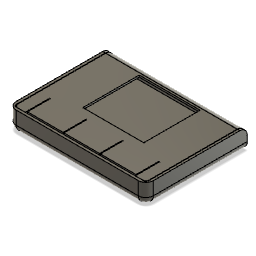
ProM Display Halter v12 (Autodesk Fusion 360 design; units mm, degrees)
Autodesk Fusion 360 part; units mm, degrees
note: some values were not read from the file. Set by a fixed rule: which sketch regions a step uses.
sketch "Skizze1" plane through (0, 0, 0) normal (0, 1, 0) x (1, 0, 0)
  line L0 (0, 0) -> (68, 0)
  line L1 (68, 0) -> (68, -48)
  line L2 (68, -48) -> (0, -48)
  line L3 (0, -48) -> (0, 0)
  line L4 (0, -48) -> (3.3, -48)
  line L5 (3.3, -48) -> (3.3, -33)
  line L6 (3.3, -33) -> (3.3, -20)
  circle A0 centre (3.3, -20) radius 2.5
  circle A1 centre (3.3, -33) radius 2.5
  line L7 (68, -48) -> (64.7, -48)
  line L8 (64.7, -48) -> (64.7, -33)
  line L9 (64.7, -33) -> (64.7, -20)
  circle A2 centre (64.7, -20) radius 2.5
  circle A3 centre (64.7, -33) radius 2.5
  dimension "d1" = 68
  dimension "d2" = 48
  dimension "d11" = 3.3
  dimension "d12" = 15
  dimension "d13" = 13
  dimension "d14" = 5
  dimension "d15" = 5
  dimension "d16" = 3.3
  dimension "d17" = 15
  dimension "d18" = 13
  dimension "d19" = 5
  dimension "d20" = 5
  constraint horizontal L0
  constraint vertical L1
  constraint horizontal L2
  constraint vertical L3
  constraint coincident L0.start L3.end
  constraint perpendicular L3 L4
  constraint perpendicular L4 L5
  constraint parallel L5 L6
  constraint coincident L6.end A0.centre
  constraint coincident L5.end L6.start
  constraint perpendicular L1 L7
  constraint vertical L8
  constraint perpendicular L2 L9
  constraint coincident L9.end A2.centre
  constraint coincident L8.end L9.start
  measures "d1" distance of L0.start L0.end
  measures "d2" distance of L0.start L2.end
  measures "d11" distance of L2.end L4.end
  measures "d12" distance of L4.end L5.end
  measures "d13" distance of L5.end L6.end
  measures "d14" diameter of A0
  measures "d15" diameter of A1
  measures "d16" distance of L1.end L7.end
  measures "d17" distance of L7.end L8.end
  measures "d18" distance of L8.end L9.end
  measures "d19" diameter of A2
  measures "d20" diameter of A3
extrude "Extrusion1" add sketch "Skizze1" along normal blind 1.2 makes body 1
move_body "Verschieben1" bodies 1 to x (1, 0, 0) y (0, 1, 0) z (0, 0, 1) at (0, 10, 0)
sketch "Skizze2" plane through (0, 0, 0) normal (0, 1, 0) x (1, 0, 0)
  line L0 (0, 0) -> (73, 0)
  line L1 (73, 0) -> (73, -54)
  line L2 (73, -54) -> (0, -54)
  line L3 (0, -54) -> (0, 0)
  dimension "d21" = 73
  dimension "d22" = 54
  constraint horizontal L0
  constraint vertical L1
  constraint horizontal L2
  constraint vertical L3
  constraint coincident L0.start L3.end
  measures "d21" distance of L0.start L0.end
  measures "d22" distance of L0.start L2.end
sketch "Skizze4" plane through (0, 0, 0) normal (0, 1, 0) x (1, 0, 0)
  line L0 (0, 0) -> (73, 0)
  line L1 (73, 0) -> (73, -54)
  line L2 (73, -54) -> (0, -54)
  line L3 (0, -54) -> (0, 0)
  line L4 (71.6, -1.4) -> (71.6, -52.6)
  line L5 (71.6, -52.6) -> (1.4, -52.6)
  line L6 (1.4, -52.6) -> (1.4, -1.4)
  line L7 (71, -2) -> (71, -52)
  line L8 (71, -52) -> (2, -52)
  line L9 (2, -52) -> (2, -2)
  line L10 (2, -2) -> (71, -2)
  line L11 (1.4, -1.4) -> (1.4, 0)
  line L12 (2, -2) -> (1.4, -2)
  line L13 (71.6, -1.4) -> (71.6, 0)
  line L14 (71, -2) -> (71.6, -2)
  line L15 (73, -24.3) -> (54, -24.3)
  line L16 (54, -24.3) -> (56.9, -24.3)
  circle A0 centre (56.9, -24.3) radius 2.9
  line L17 (56.9, -24.3) -> (56.9, 0)
  line L18 (56.9, -24.3) -> (73, -24.3)
  circle A1 centre (16.1, -24.3) radius 2.9
  line L19 (16.1, -24.3) -> (0, -24.3)
  line L20 (16.1, -24.3) -> (16.1, 0)
  line L21 (16.1, -24.3) -> (16.1, -40.5)
  circle A2 centre (16.1, -40.5) radius 2.9
  line L22 (56.9, -24.3) -> (56.9, -40.5)
  circle A3 centre (56.9, -40.5) radius 2.9
  line L23 (73, -23.8) -> (67.8, -23.8)
  line L24 (67.8, -23.8) -> (67.8, 0)
  circle A4 centre (67.8, -23.8) radius 2.5
  line L25 (67.8, -23.8) -> (67.8, -35.8)
  circle A5 centre (67.8, -35.8) radius 2.5
  line L26 (0, -23.8) -> (5.2, -23.8)
  line L27 (5.2, -23.8) -> (5.2, 0)
  circle A6 centre (5.2, -23.8) radius 2.5
  line L28 (5.2, -23.8) -> (5.2, -35.8)
  circle A7 centre (5.2, -35.8) radius 2.5
  circle A8 centre (5.2, -35.8) radius 1.4
  circle A9 centre (5.2, -23.8) radius 1.4
  circle A10 centre (67.8, -35.8) radius 1.4
  circle A11 centre (67.8, -23.8) radius 1.4
  circle A12 centre (56.9, -40.5) radius 1.1
  circle A13 centre (56.9, -24.3) radius 1.1
  circle A14 centre (16.1, -24.3) radius 1.1
  circle A15 centre (16.1, -40.5) radius 1.1
  dimension "d28" = 73
  dimension "d29" = 54
  dimension "d31" = 2
  dimension "d47" = 5.8
  dimension "d48" = 24.3
  dimension "d49" = 16.1
  dimension "d50" = 5.8
  dimension "d51" = 24.3
  dimension "d52" = 16.1
  dimension "d53" = 16.2
  dimension "d54" = 5.8
  dimension "d55" = 16.2
  dimension "d56" = 5.8
  dimension "d57" = 5.2
  dimension "d58" = 23.8
  dimension "d59" = 5
  dimension "d60" = 12
  dimension "d61" = 5
  dimension "d62" = 5.2
  dimension "d63" = 23.8
  dimension "d64" = 5
  dimension "d65" = 12
  dimension "d66" = 5
  dimension "d69" = 2.8
  dimension "d70" = 2.8
  dimension "d71" = 2.8
  dimension "d72" = 2.8
  dimension "d73" = 2.2
  dimension "d74" = 2.2
  dimension "d75" = 2.2
  dimension "d76" = 2.2
  constraint horizontal L0
  constraint vertical L1
  constraint horizontal L2
  constraint vertical L3
  constraint coincident L0.start L3.end
  constraint coincident L0 L11.end
  constraint perpendicular L0 L11
  constraint coincident L6 L12.end
  constraint perpendicular L6 L12
  constraint coincident L0 L13.end
  constraint perpendicular L0 L13
  constraint coincident L4 L14.end
  constraint perpendicular L4 L14
  constraint parallel L1 L4
  constraint parallel L2 L5
  constraint parallel L3 L6
  constraint coincident L1 L15.start
  constraint perpendicular L1 L15
  constraint parallel L15 L16
  constraint coincident L16.end A0.centre
  constraint coincident L0 L17.end
  constraint perpendicular L0 L17
  constraint coincident A1.centre L19.start
  constraint coincident L3 L19.end
  constraint perpendicular L3 L19
  constraint coincident L0 L20.end
  constraint perpendicular L0 L20
  constraint perpendicular L19 L21
  constraint coincident L21.end A2.centre
  constraint vertical L22
  constraint coincident L22.end A3.centre
  constraint coincident L1 L23.start
  constraint perpendicular L4 L23
  constraint coincident L0 L24.end
  constraint perpendicular L0 L24
  constraint coincident L23.end L24.start
  constraint perpendicular L18 L25
  constraint coincident L25.end A5.centre
  constraint coincident L3 L26.start
  constraint perpendicular L6 L26
  constraint coincident L0 L27.end
  constraint perpendicular L0 L27
  constraint coincident L26.end L27.start
  constraint perpendicular L26 L28
  constraint coincident L28.end A7.centre
  constraint concentric A7 A8
  constraint concentric A6 A9
  constraint concentric A5 A10
  constraint concentric A4 A11
  constraint concentric A3 A12
  constraint concentric A0 A13
  constraint concentric A1 A14
  constraint concentric A2 A15
  measures "d28" distance of L0.start L0.end
  measures "d29" distance of L0.start L2.end
  measures "d47" diameter of A0
  measures "d48" distance of L16.end L17.end
  measures "d49" distance of L15.start L16.end
  measures "d50" diameter of A1
  measures "d51" distance of A1.centre L20.end
  measures "d52" distance of A1.centre L19.end
  measures "d53" distance of A1.centre L21.end
  measures "d54" diameter of A2
  measures "d55" distance of L16.end L22.end
  measures "d56" diameter of A3
  measures "d57" distance of L23.start L23.end
  measures "d58" distance of L23.end L24.end
  measures "d59" diameter of A4
  measures "d60" distance of L23.end L25.end
  measures "d61" diameter of A5
  measures "d62" distance of L26.start L26.end
  measures "d63" distance of L26.end L27.end
  measures "d64" diameter of A6
  measures "d65" distance of L26.end L28.end
  measures "d66" diameter of A7
  measures "d69" diameter of A8
  measures "d70" diameter of A9
  measures "d71" diameter of A10
  measures "d72" diameter of A11
  measures "d73" diameter of A12
  measures "d74" diameter of A13
  measures "d75" diameter of A14
  measures "d76" diameter of A15
extrude "Extrusion7" add sketch "Skizze4" along normal blind 5 separate body contours L19 L27 A6 A9 | L26 L27 A6 A9 | L19 L26 A6 A9 | A1 L19 L20 A14 | A1 L20 L21 A14 | L19 A6 L28 A9 | L15 L16 A0 L17 A13 | L15 A0 L17 L18 A13 | A1 L19 L21 A14 | L19 A6 L28 A9 | L23 L24 A4 A11 | L15 L18 L24 A4 A11 | L15 A0 L18 L22 A13 | L15 L16 A0 L22 A13 | L15 L18 L23 A4 A11 | L15 L18 A4 L25 A11 | L15 L18 A4 L25 A11 | A2 | A3 | A5 | A7 makes body 2 at (59.7856, 3.3333, 24.0113) makes body 3 at (7.6876, 3.3333, 35.5511) makes body 4 at (18.9856, 3.3333, 40.2113) makes body 5 at (66.4436, 3.3333, 37.9001) makes body 6 at (59.7856, 3.3333, 40.2113) makes body 7 at (7.6876, 3.3333, 23.5511) makes body 8 at (18.9856, 3.3333, 24.0113) makes body 9 at (70.2876, 1.6667, 24.0489)
extrude "Extrusion6" add sketch "Skizze4" along normal blind 1.4 separate body contours L0 L6 L10 L11 L12 L27 | L0 L10 L20 L27 | L0 L10 L17 L20 | L0 L10 L17 L24 | L0 L4 L10 L13 L14 L24 makes body 10
extrude "Extrusion4" add sketch "Skizze4" along normal blind 2 separate body contours L9 L10 L26 L27 A6 | L10 A1 L19 L20 L27 A6 | L9 L19 L26 A6 | L7 L8 L9 L10 L15 A0 L17 L18 A1 L19 L20 A4 A6 | L19 L27 A6 A9 | L26 L27 A6 A9 | L19 L26 A6 A9 | L10 L15 A0 L17 L18 L24 A4 | A1 L19 L20 A14 | A1 L20 L21 A14 | L19 A6 L28 A9 | L7 L10 L23 L24 A4 | L15 L16 A0 L17 A13 | L15 A0 L17 L18 A13 | A1 L19 L21 A14 | L19 A6 L28 A9 | L23 L24 A4 A11 | L15 L18 L24 A4 A11 | L15 A0 L18 L22 A13 | L15 L16 A0 L22 A13 | L7 L15 L18 L23 A4 | L15 L18 L23 A4 A11 | L15 L18 A4 L25 A11 | L15 L18 A4 L25 A11 | A2 | A3 | A5 | A7 makes body 11
extrude "Extrusion3" add sketch "Skizze4" along normal blind 11 separate body contours L0 L3 L6 L11 L26 | L3 L6 L19 L26 | L1 L2 L3 L4 L5 L6 L15 L18 L19 | L1 L4 L15 L18 L23 | L0 L1 L4 L13 L23 makes body 12
extrude "Extrusion5" add sketch "Skizze4" along normal blind 9 contours L6 L9 L19 L26 | L6 L9 L12 L26 | L4 L5 L6 L7 L8 L9 L15 L18 L19 | L4 L7 L15 L18 L23 | L4 L7 L14 L23 bodies 11 12
combine "Kombinieren1" operation add target body 11 tool bodies 10
fillet "Abrundung5" radius 4 4 edges at (71, 2, 27) (71.6, 1.4, 1) (2, 2, 27) (1.4, 1.4, 1) on bodies 11
fillet "Abrundung5" radius 1 2 edges at (1.4, 10, 52.6) (71.6, 10, 52.6) on bodies 11
fillet "Abrundung6" radius 4 5 edges at (73, 0, 27) (73, 5.5, 54) (36.5, 0, 54) (0, 5.5, 54) (0, 0, 27) on bodies 11
combine "Kombinieren2" operation add target body 11 tool bodies 2 3 4 5 6 7 8 9
move_body "Verschieben2" bodies 1 to x (1, 0, 0) y (0, 1, 0) z (0, 0, 1) at (2.3776, -4.6204, 3)
sketch "Skizze8" plane through (0, 0, 0) normal (0, 1, 0) x (1, 0, 0)
  line L0 (1.4, -52.6) -> (1.4, -1.4)
  line L1 (2, -2) -> (71, -2)
  line L2 (71, -2) -> (71.6, -2)
  circle A0 centre (5.2, -35.8) radius 2
  line L3 (1.4, -1.4) -> (1.4, 0)
  circle A1 centre (5.2, -23.8) radius 2
  line L4 (71.6, -1.4) -> (71.6, -52.6)
  circle A2 centre (5.2, -35.8) radius 1.1
  circle A3 centre (5.2, -23.8) radius 1.1
  circle A4 centre (67.8, -23.8) radius 1.1
  line L5 (2, -2) -> (1.4, -2)
  line L6 (71.6, -1.4) -> (71.6, 0)
  line L7 (71.6, -52.6) -> (1.4, -52.6)
  circle A5 centre (67.8, -23.8) radius 2
  circle A6 centre (67.8, -35.8) radius 1.1
  circle A7 centre (67.8, -35.8) radius 2
  line L8 (1.4, 0) -> (71.6, 0)
  line L9 (22.4, -13) -> (50.4, -13)
  line L10 (50.4, -13) -> (50.4, -34)
  line L11 (50.4, -34) -> (22.4, -34)
  line L12 (22.4, -34) -> (22.4, -13)
  dimension "d118" = 4
  dimension "d119" = 12
  dimension "d120" = 4
  dimension "d123" = 4
  dimension "d124" = 12
  dimension "d125" = 4
  dimension "d126" = 2.2
  dimension "d127" = 2.2
  dimension "d128" = 2.2
  dimension "d129" = 2.2
  dimension "d134" = 28
  dimension "d135" = 21
  constraint coincident L5.end L0
  constraint perpendicular L0 L5
  constraint coincident L2.end L4
  constraint perpendicular L2 L4
  constraint concentric A0 A2
  constraint concentric A1 A3
  constraint concentric A6 A7
  constraint concentric A4 A5
  constraint perpendicular L6 L8
  constraint horizontal L9
  constraint vertical L10
  constraint horizontal L11
  constraint vertical L12
  measures "d118" diameter of A5
  measures "d119" distance of A4.centre A6.centre
  measures "d120" diameter of A7
  measures "d123" diameter of A1
  measures "d124" distance of A1.centre A0.centre
  measures "d125" diameter of A0
  measures "d126" diameter of A2
  measures "d127" diameter of A3
  measures "d128" diameter of A6
  measures "d129" diameter of A4
  measures "d134" distance of L9.start L9.end
  measures "d135" distance of L9.start L11.end
extrude "Extrusion14" add sketch "Skizze8" along normal blind 2 separate body contours L0 L1 L2 L4 L5 L7 | L0 L1 L2 L3 L4 L5 L6 L8 | A0 | A1 | A2 | A3 | A4 | A5 | A6 | A7 makes body 13
sketch "Skizze11" plane through (0, 0, 0) normal (0, -1, 0) x (1, 0, 0)
  line L0 (71.6, 0) -> (71.6, 52.6)
  line L1 (71.6, 52.6) -> (1.4, 52.6)
  line L2 (1.4, 52.6) -> (1.4, 0)
  line L3 (22.4, 34) -> (50.4, 34)
  line L4 (50.4, 34) -> (50.4, 13)
  line L5 (50.4, 13) -> (22.4, 13)
  line L6 (22.4, 13) -> (22.4, 34)
  line L7 (71.6, 52.6) -> (1.4, 52.6)
  line L8 (1.4, 52.6) -> (1.4, 39.6)
  line L9 (1.4, 39.6) -> (71.6, 39.6)
  line L10 (71.6, 39.6) -> (71.6, 52.6)
  line L11 (71.6, 39.6) -> (46.4, 39.6)
  line L12 (46.4, 39.6) -> (23, 39.6)
  line L13 (46.4, 39.6) -> (46, 39.6)
  line L14 (46, 39.6) -> (46, 52.6)
  line L15 (46, 52.6) -> (46.4, 52.6)
  line L16 (46.4, 52.6) -> (46.4, 39.6)
  line L17 (1.4, 39.6) -> (26.6, 39.6)
  line L18 (26.6, 39.6) -> (27, 39.6)
  line L19 (27, 39.6) -> (27, 52.6)
  line L20 (27, 52.6) -> (26.6, 52.6)
  line L21 (26.6, 52.6) -> (26.6, 39.6)
  line L22 (1.4, 0) -> (71.6, 0)
  line L23 (26.6, 39.6) -> (7.6, 39.6)
  line L24 (7.6, 39.6) -> (7.2, 39.6)
  line L25 (7.2, 39.6) -> (7.2, 52.6)
  line L26 (7.2, 52.6) -> (7.6, 52.6)
  line L27 (7.6, 52.6) -> (7.6, 39.6)
  line L28 (46.4, 39.6) -> (65.4, 39.6)
  line L29 (65.4, 39.6) -> (65.8, 39.6)
  line L30 (65.8, 39.6) -> (65.8, 52.6)
  line L31 (65.8, 52.6) -> (65.4, 52.6)
  line L32 (65.4, 52.6) -> (65.4, 39.6)
  point P0 (71.6, 52.6)
  point P1 (1.4, 52.6)
  dimension "d148" = 13
  dimension "d149" = 70.2
  dimension "d150" = 25.2
  dimension "d152" = 0.4
  dimension "d153" = 13
  dimension "d154" = 25.2
  dimension "d155" = 0.4
  dimension "d156" = 13
  dimension "d163" = 19
  dimension "d164" = 0.4
  dimension "d165" = 13
  dimension "d166" = 19
  dimension "d167" = 0.4
  dimension "d168" = 13
  constraint horizontal L7
  constraint vertical L8
  constraint horizontal L9
  constraint vertical L10
  constraint coincident P0 L0.end
  constraint perpendicular L0 L11
  constraint parallel L9 L12
  constraint horizontal L13
  constraint vertical L14
  constraint horizontal L15
  constraint vertical L16
  constraint perpendicular L2 L17
  constraint horizontal L18
  constraint vertical L19
  constraint horizontal L20
  constraint vertical L21
  constraint perpendicular L21 L23
  constraint horizontal L24
  constraint vertical L25
  constraint horizontal L26
  constraint vertical L27
  constraint perpendicular L16 L28
  constraint horizontal L29
  constraint vertical L30
  constraint horizontal L31
  constraint vertical L32
  measures "d148" distance of P0 L9.end
  measures "d149" distance of L8.end L9.end
  measures "d150" distance of L9.end L11.end
  measures "d152" distance of L11.end L13.end
  measures "d153" distance of L11.end L15.end
  measures "d154" distance of L8.end L17.end
  measures "d155" distance of L17.end L18.end
  measures "d156" distance of L17.end L20.end
  measures "d163" distance of L17.end L23.end
  measures "d164" distance of L23.end L24.end
  measures "d165" distance of L23.end L26.end
  measures "d166" distance of L11.end L28.end
  measures "d167" distance of L28.end L29.end
  measures "d168" distance of L28.end L31.end
extrude "Extrusion20" cut sketch "Skizze11" against normal blind 2 contours L1 L7 L9 L11 L29 L30 L31 L32 | L1 L7 L9 L17 L24 L25 L26 L27 bodies 13
sketch "Skizze10" plane through (0, 2, 0) normal (0, 1, 0) x (-1, 0, 0)
  line L0 (-50.4, 34) -> (-22.4, 34)
  line L1 (-22.4, 34) -> (-22.4, 13)
  line L2 (-22.4, 13) -> (-50.4, 13)
  line L3 (-50.4, 13) -> (-50.4, 34)
  line L4 (-71.6, 52.6) -> (-71.6, 0)
  line L5 (-71.6, 0) -> (-1.4, 0)
  line L6 (-1.4, 0) -> (-1.4, 52.6)
  line L7 (-65.8, 52.6) -> (-71.6, 52.6)
  line L8 (-2, 2) -> (-1.4, 2)
  line L9 (-2, 2) -> (-71, 2)
  line L10 (-71, 2) -> (-71.6, 2)
  circle A0 centre (-5.2, 23.8) radius 2
  circle A1 centre (-67.8, 23.8) radius 2
  circle A2 centre (-67.8, 35.8) radius 2
  circle A3 centre (-5.2, 35.8) radius 2
  circle A4 centre (-5.2, 35.8) radius 1.1
  circle A5 centre (-67.8, 35.8) radius 1.1
  line L11 (-1.4, 1.4) -> (-1.4, 0)
  line L12 (-1.4, 0) -> (-71.6, 0)
  line L13 (-1.4, 52.6) -> (-1.4, 1.4)
  line L14 (-71.6, 52.6) -> (-1.4, 52.6)
  line L15 (-71.6, 1.4) -> (-71.6, 52.6)
  line L16 (-71.6, 1.4) -> (-71.6, 0)
  circle A6 centre (-5.2, 23.8) radius 1.1
  circle A7 centre (-67.8, 23.8) radius 1.1
  line L17 (-1.4, 0) -> (-71.6, 0)
  line L18 (-71.6, 0) -> (-71.6, 2)
  line L19 (-71.6, 2) -> (-1.4, 2)
  line L20 (-1.4, 2) -> (-1.4, 0)
  line L21 (-1.4, 39.6) -> (-71.6, 39.6)
  line L22 (-71.6, 39.6) -> (-71.6, 39.2)
  line L23 (-71.6, 39.2) -> (-1.4, 39.2)
  line L24 (-1.4, 39.2) -> (-1.4, 39.6)
  line L25 (-65.4, 52.6) -> (-65.4, 39.6)
  line L26 (-65.4, 39.6) -> (-65.8, 39.6)
  line L27 (-65.8, 39.6) -> (-65.8, 52.6)
  line L28 (-1.4, 52.6) -> (-7.2, 52.6)
  line L29 (-7.2, 52.6) -> (-7.2, 39.6)
  line L30 (-7.2, 39.6) -> (-7.6, 39.6)
  line L31 (-7.6, 39.6) -> (-7.6, 52.6)
  line L32 (-7.6, 52.6) -> (-65.4, 52.6)
  line L33 (-65.6, 3) -> (-9.6, 3)
  line L34 (-9.6, 3) -> (-9.6, 38.5)
  line L35 (-9.6, 38.5) -> (-65.6, 38.5)
  line L36 (-65.6, 38.5) -> (-65.6, 3)
  line L37 (-65.6, 3) -> (-60.6, 3)
  line L38 (-60.6, 3) -> (-14.6, 3)
  line L39 (-14.6, 3) -> (-14.6, 38.5)
  line L40 (-14.6, 38.5) -> (-60.6, 38.5)
  line L41 (-60.6, 38.5) -> (-60.6, 3)
  line L42 (-59.6, 4) -> (-15.6, 4)
  line L43 (-15.6, 4) -> (-15.6, 37.5)
  line L44 (-15.6, 37.5) -> (-59.6, 37.5)
  line L45 (-59.6, 37.5) -> (-59.6, 4)
  line L46 (-15.6, 4) -> (-52.6, 4)
  line L47 (-52.6, 4) -> (-52.6, 37.5)
  line L48 (-15.6, 37.5) -> (-20.2, 37.5)
  line L49 (-20.2, 37.5) -> (-52.6, 37.5)
  line L50 (-52.6, 37.5) -> (-52.6, 5.1)
  line L51 (-52.6, 5.1) -> (-20.2, 5.1)
  line L52 (-52.6, 5.1) -> (-20.2, 5.1)
  line L53 (-20.2, 5.1) -> (-20.2, 35.1)
  line L54 (-20.2, 35.1) -> (-52.6, 35.1)
  line L55 (-52.6, 35.1) -> (-52.6, 5.1)
  point P0 (-1.4, 39.6)
  point P1 (-71.6, 39.6)
  dimension "d159" = 0.4
  dimension "d177" = 56
  dimension "d178" = 35.5
  dimension "d179" = 5
  dimension "d180" = 46
  dimension "d183" = -1
  dimension "d184" = 37
  dimension "d185" = 4.6
  dimension "d186" = 32.4
  dimension "d189" = 30
  constraint horizontal L17
  constraint vertical L18
  constraint horizontal L19
  constraint vertical L20
  constraint coincident L10.end L18.end
  constraint coincident L5.end L6.start
  constraint horizontal L21
  constraint vertical L22
  constraint horizontal L23
  constraint vertical L24
  constraint coincident P0 L21.start
  constraint horizontal L33
  constraint vertical L34
  constraint horizontal L35
  constraint vertical L36
  constraint perpendicular L36 L37
  constraint horizontal L38
  constraint vertical L39
  constraint horizontal L40
  constraint vertical L41
  constraint perpendicular L43 L46
  constraint coincident L44 L47.end
  constraint perpendicular L44 L47
  constraint perpendicular L43 L48
  constraint horizontal L49
  constraint vertical L50
  constraint horizontal L51
  constraint horizontal L52
  constraint vertical L53
  constraint horizontal L54
  constraint vertical L55
  measures "d159" distance of P0 L23.end
  measures "d177" distance of L33.start L33.end
  measures "d178" distance of L33.start L35.end
  measures "d179" distance of L33.start L37.end
  measures "d180" distance of L37.end L38.end
  measures "d184" distance of L42.end L46.end
  measures "d185" distance of L43.end L48.end
  measures "d186" distance of L48.end L51.end
  measures "d189" distance of L50.end L54.end
extrude "Extrusion22" cut sketch "Skizze10" against normal blind 2 contours L47 L50 L51 L52 L53 L54 L55 bodies 13
extrude "Extrusion21" cut sketch "Skizze10" against normal blind 1 contours L33 L35 L38 L39 L40 L41 | L42 L44 L45 L47 L50 L55 | L42 L43 L44 L46 L47 L48 L49 L50 L51 L52 L53 L54 | L47 L50 L51 L52 L53 L54 L55 bodies 13
extrude "Extrusion18" cut sketch "Skizze11" against normal blind 2 contours L1 L7 L9 L12 L13 L14 L15 L16 | L1 L7 L9 L12 L18 L19 L20 L21 bodies 13
extrude "Extrusion19" cut sketch "Skizze10" against normal blind 0.6 contours L4 L6 L13 L15 L21 L22 L23 L24 L26 L30 bodies 13
extrude "Extrusion17" add sketch "Skizze10" along normal blind 7.8 contours L4 L5 L6 L8 L9 L10 L11 L12 L13 L15 L16 L17 L18 L19 L20 bodies 13
extrude "Extrusion16" add sketch "Skizze10" along normal blind 4 contours A0 | A1 | A2 | A3 bodies 13
fillet "Abrundung9" radius 2 2 edges at (1.4, 1, 52.6) (71.6, 1, 52.6) on bodies 13
fillet "Abrundung10" radius 4 3 edges at (36.5, 0, 0) (71.6, 9.8, 1) (1.4, 9.8, 1) on bodies 13
fillet "Abrundung11" radius 2 1 edges at (36.5, 2, 2) on bodies 13
move_face "Flächen versetzen1" offset -0.8 3 faces at (59.0667, 0.6667, 52.6) (39.6667, 1.3333, 52.6) (20.2667, 1.3333, 52.6) on bodies 13
move_body "Verschieben3" bodies 13 to x (1, 0, 0) y (0, 1, 0) z (0, 0, 1) at (0, 11, 0)
move_body "Verschieben4" bodies 13 to x (-1, 0, 0) y (0, -1, 0) z (0, 0, 1) at (143.2, 22, 0)
move_body "Verschieben5" bodies 13 to x (1, 0, 0) y (0, 1, 0) z (0, 0, 1) at (-70, 0, 0)
fillet "Abrundung12" radius 4 2 edges at (72.3, 11, 0) (0.7, 11, 0) on bodies 11
sketch "Skizze12" plane through (0, 6.5796, 0) normal (0, 1, 0) x (-1, 0, 0)
  circle A0 centre (-67.0776, 23) radius 2.5
  circle A1 centre (-5.6776, 23) radius 2.5
  circle A2 centre (-5.6776, 36) radius 2.5
  circle A3 centre (-67.0776, 36) radius 2.5
  line L0 (-2.3776, 51) -> (-70.3776, 51)
  line L1 (-70.3776, 51) -> (-70.3776, 3)
  line L2 (-70.3776, 3) -> (-2.3776, 3)
  line L3 (-2.3776, 3) -> (-2.3776, 51)
  line L4 (-9.3776, 3) -> (-11.3776, 3)
  line L5 (-11.3776, 3) -> (-11.3776, 38)
  line L6 (-11.3776, 38) -> (-9.3776, 38)
  line L7 (-9.3776, 38) -> (-9.3776, 3)
  line L8 (-70.3776, 3) -> (-63.3776, 3)
  line L9 (-63.3776, 3) -> (-61.3776, 3)
  line L10 (-61.3776, 3) -> (-61.3776, 38)
  line L11 (-61.3776, 38) -> (-63.3776, 38)
  line L12 (-63.3776, 38) -> (-63.3776, 3)
  dimension "d190" = 2
  dimension "d191" = 35
  dimension "d194" = 2
  dimension "d195" = 35
  constraint horizontal L4
  constraint vertical L5
  constraint horizontal L6
  constraint vertical L7
  constraint coincident L2 L4.start
  constraint coincident L1.end L2.start
  constraint perpendicular L1 L8
  constraint horizontal L9
  constraint vertical L10
  constraint horizontal L11
  constraint vertical L12
  measures "d190" distance of L4.start L4.end
  measures "d191" distance of L4.start L6.end
  measures "d194" distance of L8.end L9.end
  measures "d195" distance of L8.end L11.end
extrude "Extrusion23" add sketch "Skizze12" along normal blind 1 contours L2 L4 L5 L6 L7 | L2 L9 L10 L11 L12 bodies 1
